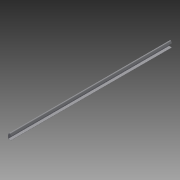
# Autodesk Inventor part: 2in rail right
Saved by Autodesk Inventor 2015 SP1 (Build 190203100, 203)
## iProperties
Created: 2015-01-12
Part Number: 2in rail right
Material: Generic
Document SubType Name: Modeling
Designer: Jarod
Density: 1 g/cm^3
Appearance: Default
Author: Jarod
Autodesk Inventor part; units mm, degrees
ref_plane "YZ Plane" through (0, 0, 0) normal (1, 0, 0) x (0, 1, 0)
ref_plane "XZ Plane" through (0, 0, 0) normal (0, 1, 0) x (-1, 0, 0)
ref_plane "XY Plane" through (0, 0, 0) normal (0, 0, 1) x (1, 0, 0)
sketch "Sketch1" plane through (0, 0, 0) normal (0, 0, 1) x (1, 0, 0)
  line L0 (0, 0) -> (-12.7, 0) construction
  line L1 (-12.7, 0) -> (-12.7, 50.8) construction
  line L2 (-12.7, 50.8) -> (0, 50.8) construction
  line L3 (0, 50.8) -> (0, 0) construction
  line L4 (-12.7, 50.8) -> (-25.4, 50.8) construction
  line L5 (-12.7, 50.8) -> (0, 50.8) construction
  line L6 (-25.4, 50.8) -> (-25.4, 0) construction
  line L7 (-25.4, 0) -> (-12.7, 0) construction
  circle A0 centre (-12.7, 6.35) radius 6.35 construction
  circle A1 centre (-12.7, 44.45) radius 6.35 construction
  line L8 (-12.7, 44.45) -> (-18.1993, 47.625) construction
  line L9 (-12.7, 44.45) -> (-6.35, 44.45) construction
  line L10 (-12.7, 44.45) -> (-7.2007, 47.625) construction
  line L11 (-12.7, 44.45) -> (-6.35, 44.45) construction
  line L12 (0, 0) -> (-25.4, 0)
  line L13 (0, 0) -> (0, -1.5875)
  line L14 (0, 0) -> (1.5875, 0) construction
  line L15 (0, -1.5875) -> (-26.9875, -1.5875)
  arc A2 (-7.2007, 47.625) -> (-18.1993, 47.625) centre (-12.7, 44.45) ccw
  line L16 (-7.2007, 47.625) -> (0, 35.153)
  line L17 (-7.2007, 47.625) -> (7.2007, 47.625) construction
  line L18 (-18.1993, 47.625) -> (-24.5493, 36.6265)
  line L19 (-18.1993, 47.625) -> (-5.4993, 47.625) construction
  line L20 (-25.4, 0) -> (-25.4, 33.4515)
  line L21 (-19.5741, 48.4187) -> (-26.1368, 37.0518)
  line L22 (-26.9875, -1.5875) -> (-26.9875, 33.8768)
  arc A3 (-26.1368, 37.0518) -> (-26.9875, 33.8768) centre (-20.6375, 33.8768) ccw
  arc A4 (-24.5493, 36.6265) -> (-25.4, 33.4515) centre (-19.05, 33.4515) ccw
  line L23 (-5.8259, 48.4187) -> (1.3748, 35.9467)
  arc A5 (-5.8259, 48.4187) -> (-19.5741, 48.4187) centre (-12.7, 44.45) ccw
  arc A6 (0, 35.153) -> (1.3748, 35.9467) centre (0.6874, 35.5498) ccw
  point P0 (-25.4, 35.153)
  dimension "d0" = 12.7
  dimension "d1" = 50.8
  dimension "d2" = 12.7
  dimension "d3" = 180
  dimension "d4" = 50.8
  dimension "d5" = 90
  dimension "d6" = 12.7
  dimension "d7" = 12.7
  dimension "d8" = 6.35
  dimension "d9" = 6.35
  dimension "d10" = 6.35
  dimension "d11" = 150
  dimension "d12" = 6.35
  dimension "d13" = 30
  dimension "d14" = 1.5875
  dimension "d15" = 90
  dimension "d16" = 26.9875
  dimension "d17" = 6.35
  dimension "d18" = 60
  dimension "d19" = 120
  dimension "d20" = 90
  dimension "d21" = 1.5875
  dimension "d22" = 6.35
  dimension "d23" = 6.35
  dimension "d24" = 1.5875
  dimension "d25" = 7.9375
  dimension "d26" = 0
  constraints: 48 end point, 10 point on circle, 8 horizontal, 7 centre point, 6 equal length, 6 point on line, 6 tangent, 4 parallel, 3 perpendicular, 2 vertical
  measures "d0" distance of L1.end L2.end
  measures "d1" distance of L0.end L1.end
  measures "d2" distance of L1.end L4.end
  measures "d3" angle of L4 L5
  measures "d4" distance of L4.end L6.end
  measures "d5" angle of L6 L4
  measures "d6" diameter of A0
  measures "d7" diameter of A1
  measures "d8" distance from line of L0 A0.centre
  measures "d9" distance from line of L2 L8.start
  measures "d10" distance of L8.start L8.end
  measures "d11" angle of L9 L8
  measures "d12" distance of L8.start L10.end
  measures "d13" angle of L11 L10
  measures "d14" distance of L0.start L13.end
  measures "d15" angle of L13 L14
  measures "d16" distance of L13.end L15.end
  measures "d17" radius of A2
  measures "d18" angle of L16 L17
  measures "d19" angle of L18 L19
  measures "d20" angle of L15 L22
  measures "d21" distance between parallel lines of L21 L18
  measures "d22" radius of A3
  measures "d23" radius of A4
  measures "d24" distance between parallel lines of L16 L23
  measures "d25" radius of A5
  measures "d26" distance of L8.start A5.centre
extrude "Extrusion1" add sketch "Sketch1" along normal blind 1524
body "Solid1"
